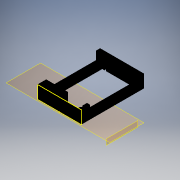
# Autodesk Inventor part: 20_Projector_Sony_Mount_1
Saved by Autodesk Inventor 2019 (Build 230136000, 136)
## iProperties
Created: 2018-08-23
Part Number: 20_Projector_Sony_Mount_1
Material: Generisch
Document SubType Name: Modeling
Designer: diederichbenedict
Density: 1 g/cm^3
Appearance: Grün - poliert
Author: diederichbenedict
Autodesk Inventor part; units mm, degrees
ref_plane "YZ Plane" through (0, 0, 0) normal (1, 0, 0) x (0, 1, 0)
ref_plane "Arbeitsebene1" through (0, 0, 0) normal (0, 0, 1) x (1, 0, 0)
sketch "Skizze1" plane through (0, 0, 0) normal (0, 0, 1) x (1, 0, 0)
  arc A0 (63.4381, 5.6873) -> (63.3881, 5.2) centre (65.7881, 5.2) ccw construction
  line L0 (63.4381, 5.6873) -> (63.4381, 7.6) construction
  line L1 (63.4381, 7.6) -> (65.7881, 7.6) construction
  arc A1 (68.1881, 5.2) -> (65.7881, 7.6) centre (65.7881, 5.2) ccw construction
  line L2 (68.1881, 5.2) -> (68.1881, -5.2) construction
  arc A2 (65.7881, -7.6) -> (68.1881, -5.2) centre (65.7881, -5.2) ccw construction
  line L3 (65.7881, -7.6) -> (63.4381, -7.6) construction
  line L4 (63.4381, -7.6) -> (63.4381, -5.6873) construction
  arc A3 (63.3881, -5.2) -> (63.4381, -5.6873) centre (65.7881, -5.2) ccw construction
  line L5 (63.3881, -5.2) -> (63.3881, 5.2) construction
  arc A4 (-72.9, 74.9) -> (-74.9, 72.9) centre (-72.9, 72.9) ccw construction
  line L6 (-74.9, 72.9) -> (-74.9, -22.9) construction
  arc A5 (-74.9, -22.9) -> (-72.9, -24.9) centre (-72.9, -22.9) ccw construction
  line L7 (-72.9, -24.9) -> (72.9, -24.9) construction
  arc A6 (72.9, -24.9) -> (74.9, -22.9) centre (72.9, -22.9) ccw construction
  line L8 (74.9, -22.9) -> (74.9, 72.9) construction
  arc A7 (74.9, 72.9) -> (72.9, 74.9) centre (72.9, 72.9) ccw construction
  line L9 (72.9, 74.9) -> (-72.9, 74.9) construction
  circle A8 centre (-70, -20) radius 1.6 construction
  circle A9 centre (70, -20) radius 1.6 construction
  circle A10 centre (70, 20) radius 1.6 construction
  circle A11 centre (-70, 20) radius 1.6 construction
  arc A12 (-58.3017, -21.066) -> (-56.7383, -21.066) centre (-57.52, -20.62) ccw construction
  line L10 (-58.3017, -21.066) -> (-67.9, -21.066) construction
  line L11 (-67.9, -21.066) -> (-67.9, -9) construction
  line L12 (-67.9, -9) -> (-64.5, -9) construction
  arc A13 (-64.5, -9) -> (-61.5, -6) centre (-64.5, -6) ccw construction
  line L13 (-61.5, -6) -> (-61.5, 6) construction
  arc A14 (-61.5, 6) -> (-64.5, 9) centre (-64.5, 6) ccw construction
  line L14 (-64.5, 9) -> (-67.9, 9) construction
  line L15 (-67.9, 28.5) -> (-67.9, 64.9) construction
  line L16 (67.9, 64.9) -> (67.9, 28.5) construction
  arc A15 (64.9, 9) -> (67.9, 12) centre (64.9, 12) ccw construction
  line L17 (64.5, 9) -> (64.9, 9) construction
  arc A16 (64.5, 9) -> (61.5, 6) centre (64.5, 6) ccw construction
  line L18 (61.5, -6) -> (61.5, 6) construction
  arc A17 (61.5, -6) -> (64.5, -9) centre (64.5, -6) ccw construction
  line L19 (64.9, -9) -> (64.5, -9) construction
  arc A18 (67.9, -12) -> (64.9, -9) centre (64.9, -12) ccw construction
  line L20 (67.9, -12) -> (67.9, -21.066) construction
  line L21 (67.9, -21.066) -> (58.3017, -21.066) construction
  arc A19 (56.7383, -21.066) -> (58.3017, -21.066) centre (57.52, -20.62) ccw construction
  line L22 (56.7383, -21.066) -> (43.0617, -21.066) construction
  arc A20 (41.4983, -21.066) -> (43.0617, -21.066) centre (42.28, -20.62) ccw construction
  line L23 (41.4983, -21.066) -> (31.1932, -21.066) construction
  arc A21 (28.8068, -21.066) -> (31.1932, -21.066) centre (30, -20) ccw construction
  line L24 (28.8068, -21.066) -> (21.1932, -21.066) construction
  arc A22 (18.8068, -21.066) -> (21.1932, -21.066) centre (20, -20) ccw construction
  line L25 (18.8068, -21.066) -> (-18.8068, -21.066) construction
  arc A23 (-21.1932, -21.066) -> (-18.8068, -21.066) centre (-20, -20) ccw construction
  line L26 (-21.1932, -21.066) -> (-28.8068, -21.066) construction
  arc A24 (-31.1932, -21.066) -> (-28.8068, -21.066) centre (-30, -20) ccw construction
  line L27 (-31.1932, -21.066) -> (-41.4983, -21.066) construction
  arc A25 (-43.0617, -21.066) -> (-41.4983, -21.066) centre (-42.28, -20.62) ccw construction
  line L28 (-43.0617, -21.066) -> (-56.7383, -21.066) construction
  arc A26 (-63.4381, -5.6873) -> (-63.3881, -5.2) centre (-65.7881, -5.2) ccw construction
  line L29 (-63.4381, -5.6873) -> (-63.4381, -7.6) construction
  line L30 (-63.4381, -7.6) -> (-65.7881, -7.6) construction
  arc A27 (-68.1881, -5.2) -> (-65.7881, -7.6) centre (-65.7881, -5.2) ccw construction
  line L31 (-68.1881, -5.2) -> (-68.1881, 5.2) construction
  arc A28 (-65.7881, 7.6) -> (-68.1881, 5.2) centre (-65.7881, 5.2) ccw construction
  line L32 (-65.7881, 7.6) -> (-63.4381, 7.6) construction
  line L33 (-63.4381, 7.6) -> (-63.4381, 5.6873) construction
  arc A29 (-63.3881, 5.2) -> (-63.4381, 5.6873) centre (-65.7881, 5.2) ccw construction
  line L34 (-63.3881, 5.2) -> (-63.3881, -5.2) construction
  arc A30 (-63.4381, -55.4873) -> (-63.3881, -55) centre (-65.7881, -55) ccw construction
  line L35 (-63.4381, -55.4873) -> (-63.4381, -57.4) construction
  line L36 (-63.4381, -57.4) -> (-65.7881, -57.4) construction
  arc A31 (-68.1881, -55) -> (-65.7881, -57.4) centre (-65.7881, -55) ccw construction
  line L37 (-68.1881, -55) -> (-68.1881, -44.6) construction
  arc A32 (-65.7881, -42.2) -> (-68.1881, -44.6) centre (-65.7881, -44.6) ccw construction
  line L38 (-65.7881, -42.2) -> (-63.4381, -42.2) construction
  line L39 (-63.4381, -42.2) -> (-63.4381, -44.1127) construction
  arc A33 (-63.3881, -44.6) -> (-63.4381, -44.1127) centre (-65.7881, -44.6) ccw construction
  line L40 (-63.3881, -44.6) -> (-63.3881, -55) construction
  arc A34 (72.9, -74.7) -> (74.9, -72.7) centre (72.9, -72.7) ccw construction
  line L41 (74.9, -72.7) -> (74.9, -26.9) construction
  arc A35 (74.9, -26.9) -> (72.9, -24.9) centre (72.9, -26.9) ccw construction
  line L42 (72.9, -24.9) -> (-72.9, -24.9) construction
  arc A36 (-72.9, -24.9) -> (-74.9, -26.9) centre (-72.9, -26.9) ccw construction
  line L43 (-74.9, -26.9) -> (-74.9, -72.7) construction
  arc A37 (-74.9, -72.7) -> (-72.9, -74.7) centre (-72.9, -72.7) ccw construction
  line L44 (-72.9, -74.7) -> (72.9, -74.7) construction
  circle A38 centre (70, -29.8) radius 1.6 construction
  circle A39 centre (-70, -29.8) radius 1.6 construction
  circle A40 centre (-70, -69.8) radius 1.6 construction
  circle A41 centre (70, -69.8) radius 1.6 construction
  arc A42 (58.3017, -28.734) -> (56.7383, -28.734) centre (57.52, -29.18) ccw construction
  line L45 (58.3017, -28.734) -> (67.9, -28.734) construction
  line L46 (67.9, -28.734) -> (67.9, -40.8) construction
  line L47 (67.9, -40.8) -> (64.5, -40.8) construction
  arc A43 (64.5, -40.8) -> (61.5, -43.8) centre (64.5, -43.8) ccw construction
  line L48 (61.5, -43.8) -> (61.5, -55.8) construction
  arc A44 (61.5, -55.8) -> (64.5, -58.8) centre (64.5, -55.8) ccw construction
  line L49 (64.5, -58.8) -> (67.9, -58.8) construction
  line L50 (67.9, -58.8) -> (67.9, -70.866) construction
  line L51 (67.9, -70.866) -> (31.1932, -70.866) construction
  arc A45 (28.8068, -70.866) -> (31.1932, -70.866) centre (30, -69.8) ccw construction
  line L52 (28.8068, -70.866) -> (21.1932, -70.866) construction
  arc A46 (18.8068, -70.866) -> (21.1932, -70.866) centre (20, -69.8) ccw construction
  line L53 (18.8068, -70.866) -> (-18.8068, -70.866) construction
  arc A47 (-21.1932, -70.866) -> (-18.8068, -70.866) centre (-20, -69.8) ccw construction
  line L54 (-21.1932, -70.866) -> (-28.8068, -70.866) construction
  arc A48 (-31.1932, -70.866) -> (-28.8068, -70.866) centre (-30, -69.8) ccw construction
  line L55 (-31.1932, -70.866) -> (-67.9, -70.866) construction
  line L56 (-67.9, -70.866) -> (-67.9, -61.8) construction
  arc A49 (-64.9, -58.8) -> (-67.9, -61.8) centre (-64.9, -61.8) ccw construction
  line L57 (-64.5, -58.8) -> (-64.9, -58.8) construction
  arc A50 (-64.5, -58.8) -> (-61.5, -55.8) centre (-64.5, -55.8) ccw construction
  line L58 (-61.5, -43.8) -> (-61.5, -55.8) construction
  arc A51 (-61.5, -43.8) -> (-64.5, -40.8) centre (-64.5, -43.8) ccw construction
  line L59 (-64.9, -40.8) -> (-64.5, -40.8) construction
  arc A52 (-67.9, -37.8) -> (-64.9, -40.8) centre (-64.9, -37.8) ccw construction
  line L60 (-67.9, -37.8) -> (-67.9, -28.734) construction
  line L61 (-67.9, -28.734) -> (-58.3017, -28.734) construction
  arc A53 (-56.7383, -28.734) -> (-58.3017, -28.734) centre (-57.52, -29.18) ccw construction
  line L62 (-56.7383, -28.734) -> (-43.0617, -28.734) construction
  arc A54 (-41.4983, -28.734) -> (-43.0617, -28.734) centre (-42.28, -29.18) ccw construction
  line L63 (-41.4983, -28.734) -> (-31.1932, -28.734) construction
  arc A55 (-28.8068, -28.734) -> (-31.1932, -28.734) centre (-30, -29.8) ccw construction
  line L64 (-28.8068, -28.734) -> (-21.1932, -28.734) construction
  arc A56 (-18.8068, -28.734) -> (-21.1932, -28.734) centre (-20, -29.8) ccw construction
  line L65 (-18.8068, -28.734) -> (18.8068, -28.734) construction
  arc A57 (21.1932, -28.734) -> (18.8068, -28.734) centre (20, -29.8) ccw construction
  line L66 (21.1932, -28.734) -> (28.8068, -28.734) construction
  arc A58 (31.1932, -28.734) -> (28.8068, -28.734) centre (30, -29.8) ccw construction
  line L67 (31.1932, -28.734) -> (41.4983, -28.734) construction
  arc A59 (43.0617, -28.734) -> (41.4983, -28.734) centre (42.28, -29.18) ccw construction
  line L68 (43.0617, -28.734) -> (56.7383, -28.734) construction
  arc A60 (63.4381, -44.1127) -> (63.3881, -44.6) centre (65.7881, -44.6) ccw construction
  line L69 (63.4381, -44.1127) -> (63.4381, -42.2) construction
  line L70 (63.4381, -42.2) -> (65.7881, -42.2) construction
  arc A61 (68.1881, -44.6) -> (65.7881, -42.2) centre (65.7881, -44.6) ccw construction
  line L71 (68.1881, -44.6) -> (68.1881, -55) construction
  arc A62 (65.7881, -57.4) -> (68.1881, -55) centre (65.7881, -55) ccw construction
  line L72 (65.7881, -57.4) -> (63.4381, -57.4) construction
  line L73 (63.4381, -57.4) -> (63.4381, -55.4873) construction
  arc A63 (63.3881, -55) -> (63.4381, -55.4873) centre (65.7881, -55) ccw construction
  line L74 (63.3881, -55) -> (63.3881, -44.6) construction
  line L75 (34.9926, -24.9) -> (-35, -24.9)
  line L76 (-35, -24.9) -> (-35, 74.9)
  line L77 (-35, 74.9) -> (34.9926, 74.9)
  line L78 (34.9926, 74.9) -> (34.9926, -24.9)
  line L79 (-67.9, 64.9) -> (-64.9, 67.9) projected
  line L80 (-64.9, 67.9) -> (64.9, 67.9) projected
  line L81 (64.9, 67.9) -> (67.9, 64.9) projected
  line L82 (-67.9, 28.5) -> (67.9, 28.5) projected
  circle A64 centre (-30, 70) radius 1.6 projected
  circle A65 centre (-70, 30) radius 1.6 projected
  circle A66 centre (20, 70) radius 1.6 projected
  circle A67 centre (70, 70) radius 1.6 projected
  circle A68 centre (70, 30) radius 1.6 projected
  circle A69 centre (30, 70) radius 1.6 projected
  circle A70 centre (-70, 70) radius 1.6 projected
  circle A71 centre (-20, 70) radius 1.6 projected
  line L83 (-67.9, 9) -> (-67.9, 21.5) projected
  line L84 (67.9, 21.5) -> (-67.9, 21.5) projected
  line L85 (67.9, 21.5) -> (67.9, 12) projected
  line L86 (-72.9, -24.9) -> (72.9, -24.9)
  point P0 (0, 0)
  point P1 (-67.9, 21.066)
  point P2 (67.9, 21.066)
  constraints: 10 end point, 2 horizontal, 2 parallel, 1 collinear, 1 point on line, 2 other
ref_plane "Arbeitsebene2" through (74.9, 24.9, 0) normal (1, 0, 0) x (0, -1, 0)
ref_plane "Arbeitsebene3" through (-73.1, -57.9, 7.2) normal (0, 0, -1) x (0, 1, 0)
extrude "Extrusion2" add sketch "Skizze1" along normal up to surface (7.2 mm away) contours L75 L76 L84 L78 | L84 L76 L82 L78 | L82 L76 L80 L78 | L80 L76 L77 L78 | A64 | A66 | A69 | A71
sketch "Skizze3" plane through (-35, -24.9, 7.2) normal (0, 0, 1) x (1, 0, 0)
  line L0 (-40.1, 14.9) -> (109.9, 14.9) construction
  line L1 (109.9, 92.2) -> (-40.1, 92.2) construction
  line L2 (0, 99.8) -> (0, 0) construction
  line L3 (0, 0) -> (69.9926, 0) construction
  line L4 (69.9926, 0) -> (69.9926, 99.8) construction
  line L5 (69.9926, 99.8) -> (0, 99.8) construction
  line L6 (69.9926, 0) -> (0, 0) construction
  line L7 (69.9926, 0) -> (0, 0) construction
  line L8 (0, 0) -> (0, 13.9) construction
  line L9 (0, 13.9) -> (69.9926, 13.9) construction
  line L10 (69.9926, 13.9) -> (69.9926, 0) construction
  line L11 (69.9926, 99.8) -> (69.9926, 0) construction
  line L12 (69.9926, 99.8) -> (0, 99.8) construction
  line L13 (0, 99.8) -> (0, 93.2) construction
  line L14 (0, 93.2) -> (69.9926, 93.2) construction
  line L15 (69.9926, 93.2) -> (69.9926, 99.8) construction
  line L16 (69.9926, 0) -> (0, 0)
  line L17 (0, 0) -> (0, 13.9)
  line L18 (0, 13.9) -> (69.9926, 13.9)
  line L19 (69.9926, 13.9) -> (69.9926, 0)
  line L20 (0, 0) -> (0, 99.8) projected
  line L21 (0, 99.8) -> (69.9926, 99.8)
  line L22 (69.9926, 99.8) -> (69.9926, 93.2)
  line L23 (69.9926, 93.2) -> (0, 93.2)
  line L24 (0, 93.2) -> (0, 99.8)
  point P0 (35, 24.9)
  dimension "d8" = 1
  dimension "d9" = 1
  constraints: 32 end point, 8 parallel, 4 horizontal, 4 perpendicular, 2 point on line
  measures "d8" distance between parallel lines of L14 L1
  measures "d9" distance between parallel lines of L0 L9
ref_plane "Arbeitsebene4" through (-73.1, -57.9, 20.3) normal (0, 0, 1) x (1, 0, 0)
extrude "Extrusion3" add sketch "Skizze3" along normal up to surface (13.1 mm away)
sketch "Skizze4" plane through (-35, -24.9, 20.3) normal (0, 0, 1) x (1, 0, 0)
  circle A0 centre (65, 4.9) radius 1.6 projected
  circle A1 centre (55, 4.9) radius 1.6 projected
  circle A2 centre (15, 4.9) radius 1.6 projected
  circle A3 centre (5, 4.9) radius 1.6 projected
  circle A4 centre (5, 94.7) radius 1.6 projected
  circle A5 centre (15, 94.7) radius 1.6 projected
  line L0 (69.9926, 0) -> (0, 0) projected
  line L1 (0, 0) -> (0, 99.8) projected
  line L2 (0, 99.8) -> (69.9926, 99.8) projected
  line L3 (69.9926, 99.8) -> (69.9926, 0) projected
  circle A6 centre (55, 94.7) radius 1.6 projected
  circle A7 centre (65, 94.7) radius 1.6 projected
  point P0 (35, 24.9)
hole "Bohrung1" at (30, -20, 20.3) at (20, -20, 20.3) at (-20, -20, 20.3) at (-30, -20, 20.3) at (30, 69.8, 20.3) at (20, 69.8, 20.3) at (-20, 69.8, 20.3) at (-30, 69.8, 20.3) direction (0, 0, -1) diameter 3.5 end through all
sketch "Skizze5" plane through (-35, -11, 7.2) normal (0, 0, 1) x (1, 0, 0)
  arc A0 (14.0986, 79.3) -> (15.9014, 79.3) centre (15, 80.8) ccw projected
  line L0 (14.0986, 79.3) -> (5.9014, 79.3) projected
  arc A1 (4.0986, 79.3) -> (5.9014, 79.3) centre (5, 80.8) ccw projected
  line L1 (4.0986, 79.3) -> (0, 79.3) projected
  line L2 (0, 79.3) -> (0, 0) projected
  line L3 (0, 0) -> (69.9926, 0) projected
  line L4 (69.9926, 0) -> (69.9926, 79.3) projected
  line L5 (69.9926, 79.3) -> (65.9014, 79.3) projected
  arc A2 (64.0986, 79.3) -> (65.9014, 79.3) centre (65, 80.8) ccw projected
  line L6 (64.0986, 79.3) -> (55.9014, 79.3) projected
  arc A3 (54.0986, 79.3) -> (55.9014, 79.3) centre (55, 80.8) ccw projected
  line L7 (54.0986, 79.3) -> (15.9014, 79.3) projected
  line L8 (0, 0) -> (69.9926, 0) projected
  line L9 (14.0986, 79.3) -> (5.9014, 79.3) projected
  line L10 (60, 0) -> (10, 0)
  line L11 (10, 0) -> (10, 79.3)
  line L12 (10, 79.3) -> (60, 79.3)
  line L13 (60, 79.3) -> (60, 0)
  point P0 (35, 11)
  constraints: 8 end point, 2 parallel, 1 horizontal, 1 midpoint, 1 perpendicular, 1 point on line
extrude "Extrusion4" cut sketch "Skizze5" against normal blind 10 contours L12 A0 | A0 L7 A3 L6 L13 L3 L11 L0 | L12 A3
sketch "Skizze6" plane through (-35, -24.9, 0) normal (0, -1, 0) x (1, 0, 0)
  line L0 (0, 0) -> (0, 20.3) projected
  line L1 (69.9926, 0) -> (0, 0) projected
  line L2 (69.9926, 0) -> (69.9926, 20.3) projected
  line L3 (69.9926, 20.3) -> (0, 20.3) projected
  point P0 (35, 0)
sketch "Skizze7" plane through (-35, -24.9, 0) normal (0, -1, 0) x (1, 0, 0)
  line L0 (74.9, 16.6407) -> (96.8, 16.6407) construction
  line L1 (74.9, 9.8533) -> (74.9, 16.6407) construction
  line L2 (96.8, 9.8533) -> (74.9, 9.8533) construction
  line L3 (96.8, 16.6407) -> (96.8, 9.8533) construction
  line L4 (39.9, 9.8533) -> (39.9, 16.6407) construction
  line L5 (39.9, 16.6407) -> (59.9, 16.6407) construction
  line L6 (59.9, 9.8533) -> (39.9, 9.8533) construction
  line L7 (0, 0) -> (0, 20.3) construction
  line L8 (69.9926, 0) -> (0, 0) construction
  line L9 (69.9926, 0) -> (69.9926, 20.3) construction
  line L10 (69.9926, 20.3) -> (0, 20.3) construction
  line L11 (59.9, 16.6407) -> (59.9, 9.8533) construction
  line L12 (34.8554, 6.194) -> (64.9446, 6.194)
  line L13 (64.9446, 6.194) -> (64.9446, 20.3)
  line L14 (64.9446, 20.3) -> (34.8554, 20.3)
  line L15 (34.8554, 20.3) -> (34.8554, 6.194)
  line L16 (34.8554, 6.194) -> (64.9446, 20.3) construction
  line L17 (64.9446, 6.194) -> (34.8554, 20.3) construction
  point P0 (35, 0)
  point P1 (49.9, 13.247)
  constraints: 12 end point, 2 midpoint, 2 parallel, 1 horizontal, 1 perpendicular, 1 point on line
extrude "Extrusion5" cut sketch "Skizze7" against normal blind 20
